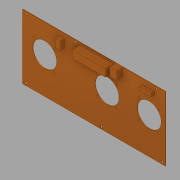
# Autodesk Inventor part: PCB
Saved by Autodesk Inventor 2017 (Build 210142000, 142)
## iProperties
Created: 2021-05-31
Part Number: PCB
Material: Gold
Document SubType Name: Modeling
Designer: Win240
Density: 19.3 g/cm^3
Appearance: Metal 1600F Hot
Mass: 2280.05 g
Surface Area: 1063.05 cm^2
Volume: 118.137 cm^3
Author: Win240
Autodesk Inventor part; units mm, degrees
ref_plane "YZ Plane" through (0, 0, 0) normal (1, 0, 0) x (0, 1, 0)
sketch "Sketch1" plane through (0, 0, 0) normal (0, 0, 1) x (1, 0, 0)
  line L0 (-177.5, -80) -> (177.5, -80)
  line L1 (177.5, -80) -> (177.5, 80)
  line L2 (177.5, 80) -> (-177.5, 80)
  line L3 (-177.5, 80) -> (-177.5, -80)
  line L4 (-177.5, -80) -> (177.5, 80) construction
  line L5 (177.5, -80) -> (-177.5, 80) construction
  circle A0 centre (-122.5, 10) radius 30
  circle A1 centre (32.5, 10) radius 30
  circle A2 centre (137.5, 10) radius 30
  line L6 (-152.5, 80) -> (-152.5, -80) construction
  line L7 (2.5, 80) -> (2.5, -80) construction
  line L8 (107.5, -80) -> (107.5, 80) construction
  line L9 (-177.5, -20) -> (177.5, -20) construction
  line L10 (-147.5, -15) -> (-97.5, -15) construction
  line L11 (-97.5, -15) -> (-97.5, 35) construction
  line L12 (-97.5, 35) -> (-147.5, 35) construction
  line L13 (-147.5, 35) -> (-147.5, -15) construction
  line L14 (-147.5, -15) -> (-97.5, 35) construction
  line L15 (-97.5, -15) -> (-147.5, 35) construction
  line L16 (7.5, -15) -> (57.5, -15) construction
  line L17 (57.5, -15) -> (57.5, 35) construction
  line L18 (57.5, 35) -> (7.5, 35) construction
  line L19 (7.5, 35) -> (7.5, -15) construction
  line L20 (7.5, -15) -> (57.5, 35) construction
  line L21 (57.5, -15) -> (7.5, 35) construction
  line L22 (112.5, -15) -> (162.5, -15) construction
  line L23 (162.5, -15) -> (162.5, 35) construction
  line L24 (162.5, 35) -> (112.5, 35) construction
  line L25 (112.5, 35) -> (112.5, -15) construction
  line L26 (112.5, -15) -> (162.5, 35) construction
  line L27 (162.5, -15) -> (112.5, 35) construction
  circle A3 centre (-147.5, 35) radius 2.25
  circle A4 centre (-97.5, 35) radius 2.25
  circle A5 centre (-97.5, -15) radius 2.25
  circle A6 centre (-147.5, -15) radius 2.25
  circle A7 centre (7.5, 35) radius 2.25
  circle A8 centre (57.5, 35) radius 2.25
  circle A9 centre (57.5, -15) radius 2.25
  circle A10 centre (7.5, -15) radius 2.25
  circle A11 centre (112.5, 35) radius 2.25
  circle A12 centre (162.5, 35) radius 2.25
  circle A13 centre (162.5, -15) radius 2.25
  circle A14 centre (112.5, -15) radius 2.25
  point P0 (0, 0)
  dimension "d0" = 160
  dimension "d1" = 355
  dimension "d4" = 25
  dimension "d6" = 180
  dimension "d8" = 285
  dimension "d9" = 100
  dimension "d10" = 60
  dimension "d11" = 50
  dimension "d12" = 4.5
  constraints: 56 end point, 15 centre point, 13 equal radius, 12 coincident, 8 midpoint, 8 parallel, 8 point on line, 6 tangent, 5 equal length, 5 horizontal, 4 perpendicular, 3 vertical
  measures "d0" distance of L0.end L1.end
  measures "d1" distance of L1.end L2.end
  measures "d4" distance between parallel lines of L3 L6
  measures "d6" distance between parallel lines of L3 L7
  measures "d8" distance between parallel lines of L8 L3
  measures "d9" distance between parallel lines of L9 L2
  measures "d10" diameter of A0
  measures "d11" distance of L11.end L12.end
  measures "d12" diameter of A3
extrude "PCB" add sketch "Sketch1" along normal blind 1.6
ref_plane "Work Plane1" through (0, 0, 2.6) normal (0, 0, 1) x (1, 0, 0)
ref_plane "Work Plane2" through (0, 0, 13.6) normal (0, 0, 1) x (1, 0, 0)
sketch "Sketch2" plane through (0, 0, 1.6) normal (0, 0, 1) x (1, 0, 0)
  line L0 (-177.5, 80) -> (-177.5, -80) construction
  line L1 (177.5, 80) -> (-177.5, 80) construction
  line L2 (-83.5, 71) -> (-71.5, 71)
  line L3 (-71.5, 71) -> (-71.5, 50)
  line L4 (-71.5, 50) -> (-83.5, 50)
  line L5 (-83.5, 50) -> (-83.5, 71)
  point P0 (0, 0)
  dimension "d15" = 94
  dimension "d16" = 106
  dimension "d17" = 9
  dimension "d18" = 30
  constraints: 8 end point, 2 parallel, 1 horizontal, 1 perpendicular
  measures "d15" distance between parallel lines of L0 L5
  measures "d16" distance between parallel lines of L3 L0
  measures "d17" distance between parallel lines of L1 L2
  measures "d18" distance between parallel lines of L1 L4
extrude "USB" add sketch "Sketch2" against normal up to surface (11 mm away) from surface at 12
sketch "Sketch3" plane through (0, 0, 1.6) normal (0, 0, 1) x (1, 0, 0)
  line L0 (-32.5, 76) -> (49.5, 76)
  line L1 (49.5, 76) -> (49.5, 58)
  line L2 (49.5, 58) -> (-32.5, 58)
  line L3 (-32.5, 58) -> (-32.5, 76)
  line L4 (-177.5, 80) -> (-177.5, -80) construction
  line L5 (177.5, 80) -> (-177.5, 80) construction
  point P0 (0, 0)
  dimension "d21" = 145
  dimension "d22" = 227
  dimension "d23" = 4
  dimension "d24" = 22
  constraints: 8 end point, 2 parallel, 1 horizontal, 1 perpendicular
  measures "d21" distance between parallel lines of L3 L4
  measures "d22" distance between parallel lines of L1 L4
  measures "d23" distance between parallel lines of L0 L5
  measures "d24" distance between parallel lines of L2 L5
extrude "Extrusion3" add sketch "Sketch3" along normal blind 21
sketch "Sketch4" plane through (0, 0, 1.6) normal (0, 0, 1) x (1, 0, 0)
  line L0 (122.5, 68) -> (151.5, 68)
  line L1 (151.5, 68) -> (151.5, 60)
  line L2 (151.5, 60) -> (122.5, 60)
  line L3 (122.5, 60) -> (122.5, 68)
  line L4 (177.5, -80) -> (177.5, 80) construction
  line L5 (177.5, 80) -> (-177.5, 80) construction
  point P0 (0, 0)
  dimension "d27" = 26
  dimension "d28" = 55
  dimension "d29" = 12
  dimension "d30" = 20
  constraints: 8 end point, 2 parallel, 1 horizontal, 1 perpendicular
  measures "d27" distance between parallel lines of L4 L1
  measures "d28" distance between parallel lines of L3 L4
  measures "d29" distance between parallel lines of L5 L0
  measures "d30" distance between parallel lines of L2 L5
extrude "Extrusion4" add sketch "Sketch4" along normal blind 9
sketch "Sketch5" plane through (0, 0, 1.6) normal (0, 0, 1) x (1, 0, 0)
  line L0 (177.5, 80) -> (-177.5, 80) projected
  line L1 (71.5, 80) -> (71.5, 59.3001)
  line L2 (71.5, 59.3001) -> (54.5, 59.3001)
  line L3 (54.5, 59.3001) -> (54.5, 80)
  point P0 (0, 0)
  dimension "d33" = 249
  dimension "d34" = 232
  constraints: 6 end point, 2 point on line, 2 vertical, 1 horizontal
  measures "d33" distance from line of L0.end L1
  measures "d34" distance from line of L0.end L3
extrude "Extrusion5" add sketch "Sketch5" along normal blind 15
sketch "Sketch6" plane through (0, 0, 1.6) normal (0, 0, 1) x (1, 0, 0)
  line L0 (54.5, 80) -> (-177.5, 80) projected
  line L1 (-177.5, 80) -> (-177.5, -80) projected
  line L2 (-177.5, -80) -> (177.5, -80) projected
  line L3 (177.5, -80) -> (177.5, 80) projected
  line L4 (177.5, 80) -> (71.5, 80) projected
  circle A0 centre (169.5, -75) radius 3
  circle A1 centre (18.5, -75) radius 3
  circle A2 centre (155.5, 74) radius 3
  circle A3 centre (-47.5, 74) radius 3
  circle A4 centre (-169.5, -75) radius 3
  circle A5 centre (-169.5, 74) radius 3
  line L5 (-169.5, 74) -> (-47.5, 74) construction
  line L6 (-47.5, 74) -> (155.5, 74) construction
  line L7 (169.5, -75) -> (18.5, -75) construction
  line L8 (18.5, -75) -> (-169.5, -75) construction
  point P0 (0, 0)
  dimension "d37" = 6
  dimension "d38" = 8
  dimension "d39" = 196
  dimension "d40" = 347
  dimension "d41" = 8
  dimension "d42" = 130
  dimension "d43" = 333
  dimension "d44" = 6
  dimension "d45" = 5
  constraints: 8 end point, 6 centre point, 5 equal radius, 4 horizontal
  measures "d37" diameter of A2
  measures "d38" distance from line of L8.end L1
  measures "d39" distance from line of L7.end L1
  measures "d40" distance from line of L1 L7.start
  measures "d41" distance from line of L5.start L1
  measures "d42" distance from line of L5.end L1
  measures "d43" distance from line of L6.end L1
  measures "d44" distance between parallel lines of L0 L5
  measures "d45" distance between parallel lines of L2 L8
extrude "Extrusion6" cut sketch "Sketch6" against normal up to surface (1.6 mm away)
body "Solid1"
